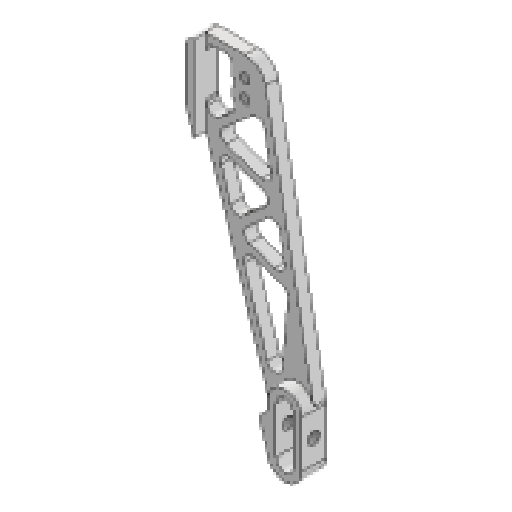
# Autodesk Inventor part: VerticalSlideMiddleTop2.2
Saved by Autodesk Inventor 2023 (Build 270158000, 158)
## iProperties
Created: 2022-10-14
Part Number: VerticalSlideMiddleTop2.2
Material: Generic
Document SubType Name: Modeling
Designer: deli
Density: 1 g/cm^3
Appearance: Default
Mass: 2.31146 g
Surface Area: 29.6295 cm^2
Volume: 2.31146 cm^3
Author: deli
Autodesk Inventor part; units mm, degrees
ref_plane "YZ Plane" through (0, 0, 0) normal (1, 0, 0) x (0, 1, 0)
ref_plane "XZ Plane" through (0, 0, 0) normal (0, 1, 0) x (-1, 0, 0)
ref_plane "XY Plane" through (0, 0, 0) normal (0, 0, 1) x (1, 0, 0)
sketch "Sketch1" plane through (0, 0, 0) normal (0, 0, 1) x (1, 0, 0)
  line L0 (-75.1619, -110.5247) -> (-75.1619, -123.5247)
  line L1 (-75.0706, -124.1221) -> (-53.9679, -191.5442)
  circle A0 centre (-63.1619, -118.2747) radius 1.25
  circle A1 centre (-63.1619, -113.7747) radius 1.25
  arc A2 (-52.1619, -190.2747) -> (-47.6619, -190.2747) centre (-49.9119, -190.2747) ccw
  arc A3 (-47.6619, -178.2747) -> (-52.1619, -178.2747) centre (-49.9119, -178.2747) ccw
  line L2 (-47.6619, -178.2747) -> (-47.6619, -190.2747)
  line L3 (-52.1619, -178.2747) -> (-52.1619, -190.2747)
  line L4 (-45.6619, -178.2747) -> (-45.6619, -190.2747)
  arc A4 (-53.9679, -191.5442) -> (-45.6619, -190.2747) centre (-49.9119, -190.2747) ccw
  arc A5 (-45.6619, -178.2747) -> (-45.7364, -177.4828) centre (-49.9119, -178.2747) ccw
  line L5 (-45.7364, -177.4828) -> (-58.0039, -112.7965)
  line L6 (-73.1619, -108.5247) -> (-63.1619, -108.5247)
  arc A6 (-58.0039, -112.7965) -> (-63.1619, -108.5247) centre (-63.1619, -113.7747) ccw
  arc A7 (-73.1619, -108.5247) -> (-75.1619, -110.5247) centre (-73.1619, -110.5247) ccw
  arc A8 (-75.1619, -123.5247) -> (-75.0706, -124.1221) centre (-73.1619, -123.5247) ccw
  line L7 (-52.1619, -182.7747) -> (-56.1619, -182.7747)
  line L8 (-56.1619, -182.7747) -> (-56.1619, -185.7747)
  line L9 (-56.1619, -185.7747) -> (-52.1619, -185.7747)
  point P0 (0, 0)
  dimension "d2" = 2.5
  dimension "d11" = 2
  dimension "d22" = 12
  dimension "d46" = 2
  dimension "d47" = 4.5
  dimension "d84" = 4
  dimension "d86" = 12
  dimension "d87" = 12
  dimension "d88" = 23
  dimension "d90" = 4
  dimension "d91" = 3
  dimension "d92" = 4.5
  dimension "d94" = 15
  dimension "d96" = 2
  dimension "d147" = 72
  constraints: 20 end point, 16 point on circle, 13 tangent, 9 centre point, 4 equal radius, 4 point on line, 3 perpendicular, 2 coincident, 2 vertical, 1 concentric, 1 horizontal, 1 parallel
  measures "d2" diameter of A0
  measures "d22" distance of A2.centre A3.centre
  measures "d46" radial gap between concentric circles of A4 A2
  measures "d47" distance between parallel lines of L2 L3
  measures "d84" distance edge to line of A1 L6
  measures "d86" distance from line of A1.centre L0
  measures "d87" distance from line of A0.centre L0
  measures "d88" distance between parallel lines of L3 L0
  measures "d90" distance of L7.start L7.end
  measures "d91" distance of L7.end L8.end
  measures "d92" distance from line of L3.start L7
  measures "d94" distance from line of L6 L0.end
  measures "d96" radius of A7
  measures "d147" vertical distance of A2.centre A0.centre
extrude "Extrusion1" add sketch "Sketch1" along normal blind 6.35 contours A7 L6 A6 L5 A5 L4 A4 L1 L9 L3 A2 L2 A3 L7 L8 A8 L0 | L8 L7 L3 L9 L1
thread "Thread2" size "M3x0.5" class "6H" standard "ANSI Metric M Profile" full length
thread "Thread6" size "M3x0.5" class "6H" standard "ANSI Metric M Profile" full length
sketch "Sketch12" plane through (0, 0, 6.35) normal (0, 0, 1) x (1, 0, 0)
  line L0 (-75.1619, -110.5247) -> (-75.1619, -123.5247) projected
  arc A0 (-75.1619, -123.5247) -> (-75.0706, -124.1221) centre (-73.1619, -123.5247) ccw projected
  line L1 (-75.0706, -124.1221) -> (-53.9679, -191.5442) projected
  arc A1 (-53.9679, -191.5442) -> (-45.6619, -190.2747) centre (-49.9119, -190.2747) ccw projected
  line L2 (-45.6619, -190.2747) -> (-45.6619, -178.2747) projected
  arc A2 (-45.6619, -178.2747) -> (-45.7364, -177.4828) centre (-49.9119, -178.2747) ccw projected
  line L3 (-45.7364, -177.4828) -> (-58.0039, -112.7965) projected
  arc A3 (-58.0039, -112.7965) -> (-63.1619, -108.5247) centre (-63.1619, -113.7747) ccw projected
  line L4 (-63.1619, -108.5247) -> (-73.1619, -108.5247) projected
  arc A4 (-73.1619, -108.5247) -> (-75.1619, -110.5247) centre (-73.1619, -110.5247) ccw projected
  circle A5 centre (-63.1619, -118.2747) radius 1.25 projected
  circle A6 centre (-63.1619, -113.7747) radius 1.25 projected
  line L5 (-47.6619, -178.2747) -> (-47.6619, -190.2747) projected
  arc A7 (-52.1619, -190.2747) -> (-47.6619, -190.2747) centre (-49.9119, -190.2747) ccw projected
  line L6 (-52.1619, -190.2747) -> (-52.1619, -178.2747) projected
  arc A8 (-47.6619, -178.2747) -> (-52.1619, -178.2747) centre (-49.9119, -178.2747) ccw projected
  line L7 (-73.1619, -123.5247) -> (-73.1619, -110.5247)
  line L8 (-73.1619, -110.5247) -> (-63.1619, -110.5247)
  line L9 (-59.9689, -113.1691) -> (-48.3732, -174.313)
  line L10 (-54.1619, -184.2287) -> (-73.1619, -123.5247)
  line L11 (-54.1619, -178.2747) -> (-54.1619, -184.2287)
  arc A9 (-65.5072, -116.0247) -> (-60.8167, -116.0247) centre (-63.1619, -118.2747) ccw
  arc A10 (-63.1619, -110.5247) -> (-65.5072, -116.0247) centre (-63.1619, -113.7747) ccw
  arc A11 (-60.8167, -116.0247) -> (-59.9689, -113.1691) centre (-63.1619, -113.7747) ccw
  arc A12 (-48.3732, -174.313) -> (-54.1619, -178.2747) centre (-49.9119, -178.2747) ccw
  line L12 (-58.8857, -118.8808) -> (-71.2754, -129.5521)
  line L13 (-55.8389, -134.9463) -> (-71.2754, -129.5521)
  line L14 (-71.9261, -127.473) -> (-64.6193, -121.1796)
  line L15 (-54.93, -181.7747) -> (-52.1619, -181.7747)
  line L16 (-52.1619, -190.2747) -> (-52.1619, -178.2747) projected
  line L17 (-70.5309, -131.9309) -> (-55.4086, -137.2152)
  line L18 (-66.017, -146.3523) -> (-55.4086, -137.2152)
  line L19 (-65.3663, -148.4314) -> (-54.9783, -139.4842)
  line L20 (-65.3663, -148.4314) -> (-52.4238, -152.954)
  line L21 (-54.6102, -182.7966) -> (-51.9935, -155.223)
  line L22 (-64.6217, -150.8102) -> (-51.9935, -155.223)
  point P0 (0, 0)
  point P1 (-54.1619, -181.7747)
  point P2 (-61.041, -120.7372)
  point P3 (-54.5132, -181.7747)
  dimension "d156" = 2
  dimension "d159" = 2
  dimension "d161" = 2
  dimension "d162" = 2
  dimension "d163" = 2
  dimension "d164" = 2
  dimension "d165" = 2
  dimension "d166" = 2
  dimension "d167" = 60
  dimension "d168" = 60
  dimension "d172" = 2
  dimension "d173" = 3.5
  dimension "d175" = 2
  dimension "d177" = 2
  dimension "d178" = 2
  constraints: 29 end point, 9 point on circle, 7 point on line, 6 parallel, 4 centre point, 2 tangent, 1 perpendicular, 12 other
  measures "d156" distance between parallel lines of L0 L7
  measures "d159" radial gap between concentric circles of A5 A9
  measures "d161" radial gap between concentric circles of A10 A6
  measures "d162" radial gap between concentric circles of A11 A6
  measures "d163" distance between parallel lines of L3 L9
  measures "d164" radial gap between concentric circles of A12 A8
  measures "d165" distance between parallel lines of L6 L11
  measures "d167" angle of L9 L12
  measures "d168" angle of L13 L12
  measures "d172" distance between parallel lines of L12 L14
  measures "d173" distance from line of A2.centre L15
  measures "d175" distance between parallel lines of L13 L17
  measures "d177" distance between parallel lines of L19 L18
  measures "d178" distance between parallel lines of L20 L22
extrude "Extrusion10" cut sketch "Sketch12" against normal blind 10 contours L7 L8 A10 A9 L14 L10 | L12 L9 L13 | L17 L18 L10 | L19 L9 L20 | L22 L21 L15 L10
fillet "Fillet6" radius 2 19 edges at (-73.1619, -110.5247, 3.175) (-63.1619, -110.5247, 3.175) (-65.5072, -116.0247, 3.175) (-64.6193, -121.1796, 3.175) (-71.9261, -127.473, 3.175) (-73.1619, -123.5247, 3.175) (-71.2754, -129.5521, 3.175) (-58.8857, -118.8808, 3.175) (-55.8389, -134.9463, 3.175) (-70.5309, -131.9309, 3.175) (-66.017, -146.3523, 3.175) (-55.4086, -137.2152, 3.175) (-65.3663, -148.4314, 3.175) (-54.9783, -139.4842, 3.175) (-52.4238, -152.954, 3.175) (-51.9935, -155.223, 3.175) (-64.6217, -150.8102, 3.175) (-54.5132, -181.7747, 3.175) (-54.93, -181.7747, 3.175)
sketch "Sketch13" plane through (0, 0, 6.35) normal (0, 0, 1) x (1, 0, 0)
  line L0 (-73.1619, -104.5087) -> (-54.1107, -104.5087)
  line L1 (-54.1619, -181.7747) -> (-73.1619, -181.7747)
  line L2 (-73.1619, -181.7747) -> (-73.1619, -104.5087)
  line L3 (-75.1619, -110.5247) -> (-75.1619, -123.5247) projected
  arc A0 (-47.6619, -178.2747) -> (-52.1619, -178.2747) centre (-49.9119, -178.2747) ccw projected
  line L4 (-52.1619, -190.2747) -> (-52.1619, -178.2747) projected
  line L5 (-56.7677, -143.7571) -> (-60.2863, -148.1457) projected
  line L6 (-45.7364, -177.4828) -> (-58.0039, -112.7965) projected
  line L7 (-54.1619, -190.2747) -> (-54.1619, -178.2747)
  arc A1 (-45.6619, -178.2747) -> (-54.1619, -178.2747) centre (-49.9119, -178.2747) ccw
  line L8 (-58.0039, -112.7965) -> (-54.1107, -104.5087)
  point P0 (0, 0)
  point P1 (-45.7364, -177.4828)
  dimension "d134" = 2
  dimension "d135" = 3.5
  dimension "d155" = 2
  constraints: 10 end point, 2 point on circle, 1 centre point, 1 horizontal, 1 parallel, 1 other
  measures "d134" distance between parallel lines of L3 L2
  measures "d135" distance from line of A0.centre L1
  measures "d155" distance between parallel lines of L4 L7
extrude "Extrusion11" cut sketch "Sketch13" against normal blind 3.175
fillet "Fillet11" radius 2 2 edges at (-57.0257, -181.7747, 4.7625) (-54.1619, -181.7747, 4.7625)
sketch "Sketch8" plane through (-52.1619, -190.2747, 0) normal (1, 0, 0) x (0, 0, -1)
  line L0 (0, 0) -> (0, 12) construction
  line L1 (0, 12) -> (-6.35, 12) construction
  line L2 (-6.35, 0) -> (-6.35, 12) construction
  line L3 (0, 0) -> (-6.35, 0) construction
  line L4 (0, 0) -> (-6.35, 0) construction
  line L5 (-6.35, 12) -> (0, 0) construction
  line L6 (-6.35, 0) -> (0, 12) construction
  circle A0 centre (-3.175, 6) radius 1.5
  point P0 (0, 190.2747)
  dimension "d97" = 3
  constraints: 4 end point, 1 centre point, 1 midpoint
  measures "d97" diameter of A0
extrude "Extrusion13" cut sketch "Sketch8" along normal blind 10 and the other way blind 5
thread "Thread7" size "M3x0.5" class "6H" standard "ANSI Metric M Profile" full length
thread "Thread8" size "M3x0.5" class "6H" standard "ANSI Metric M Profile" full length
equation "\"d22\" = d17"
equation "\"d17\" = 12"
body "Solid1"
